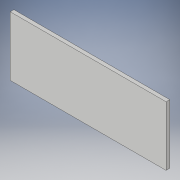
# Autodesk Inventor part: short top side 5.25x2
Saved by Autodesk Inventor 2017 (Build 210142000, 142)
## iProperties
Created: 2017-03-02
Part Number: short top side 5.25x2
Material: Generic
Document SubType Name: Modeling
Designer: Jess
Density: 1 g/cm^3
Appearance: Default
Author: Jess
Autodesk Inventor part; units mm, degrees
ref_plane "YZ Plane" through (0, 0, 0) normal (1, 0, 0) x (0, 1, 0)
ref_plane "XZ Plane" through (0, 0, 0) normal (0, 1, 0) x (-1, 0, 0)
ref_plane "XY Plane" through (0, 0, 0) normal (0, 0, 1) x (1, 0, 0)
sketch "Sketch1" plane through (0, 0, 0) normal (0, 0, 1) x (1, 0, 0)
  line L0 (-16.3863, 6.9761) -> (116.9637, 6.9761)
  line L1 (116.9637, 6.9761) -> (116.9637, -43.8239)
  line L2 (116.9637, -43.8239) -> (-16.3863, -43.8239)
  line L3 (-16.3863, -43.8239) -> (-16.3863, 6.9761)
  point P0 (0, 0)
  dimension "d0" = 133.35
  dimension "d1" = 50.8
  constraints: 8 end point, 2 parallel, 1 horizontal, 1 perpendicular
  measures "d0" distance of L1.end L2.end
  measures "d1" distance of L0.end L1.end
extrude "Extrusion1" add sketch "Sketch1" along normal blind 3.175
body "Solid1"
